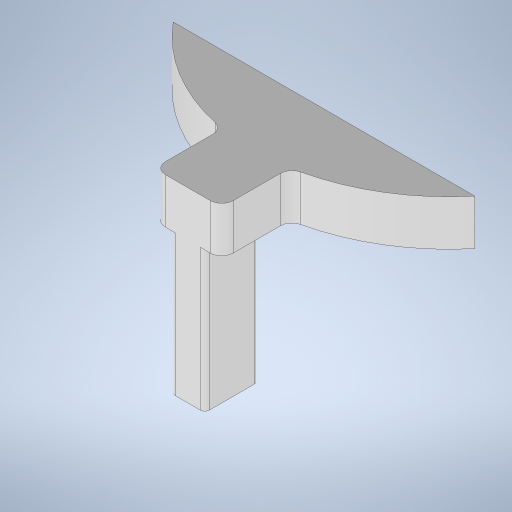
# Autodesk Inventor part: zigu1
Saved by Autodesk Inventor 2024.3 (Build 283343010, 343A)
## iProperties
Created: 2025-10-17
Part Number: zigu1
Material: 一般
Document SubType Name: Modeling
Designer: tanoue_kota
Density: 1 g/cm^3
Appearance: 既定
Author: tanoue_kota
Autodesk Inventor part; units mm, degrees
ref_plane "YZ Plane" through (0, 0, 0) normal (1, 0, 0) x (0, 1, 0)
ref_plane "XZ Plane" through (0, 0, 0) normal (0, 1, 0) x (-1, 0, 0)
ref_plane "XY Plane" through (0, 0, 0) normal (0, 0, 1) x (1, 0, 0)
sketch "スケッチ1" plane through (0, 0, 0) normal (0, 1, 0) x (-1, 0, 0)
  circle A0 centre (0, 0) radius 86.2565
  line L0 (0, 0) -> (86.2565, 0)
  line L1 (66.4468, 55) -> (-66.4468, 55)
  line L2 (0, 55) -> (14.9, 55)
  line L3 (14.9, 55) -> (14.9, 115)
  line L4 (14.9, 115) -> (0, 115)
  line L5 (0, 115) -> (0, 55)
  line L6 (-14.9, 55) -> (-14.9, 115)
  line L7 (-14.9, 115) -> (0, 115)
  point P0 (14.9, 84.9598)
  point P1 (-14.9, 84.9598)
  dimension "d0" = 172.513
  dimension "d1" = 55
  dimension "d2" = 14.9
  dimension "d3" = 60
  constraints: 16 end point, 3 parallel, 3 point on circle, 2 horizontal, 2 symmetric about line, 1 centre point, 1 coincident, 1 midpoint, 1 perpendicular
  measures "d0" diameter of A0
  measures "d1" distance between parallel lines of L0 L1
  measures "d2" distance between parallel lines of L5 L3
  measures "d3" distance between parallel lines of L1 L4
extrude "押し出し1" add sketch "スケッチ1" along normal blind 20 contours L1 L3 A0 | A0 L6 L1 | L3 L1 L5 A0 | A0 L5 L4 L3 | L6 L7 L5 A0 | A0 L5 L1 L6
sketch "スケッチ2" plane through (0, 0, 0) normal (0, -1, 0) x (1, 0, 0)
  arc A0 (66.4468, 55) -> (14.9, 84.9598) centre (0, 0) ccw projected
  circle A1 centre (0, 0) radius 86.2565
  line L0 (-14.9, 115) -> (14.9, 115) projected
  line L1 (0, 115) -> (7.475, 115)
  line L2 (7.475, 115) -> (7.475, 91.2565)
  line L3 (7.475, 91.2565) -> (0, 91.2565)
  line L4 (0, 91.2565) -> (0, 115)
  line L5 (-7.475, 115) -> (-7.475, 91.2565)
  line L6 (-7.475, 91.2565) -> (0, 91.2565)
  line L7 (14.9, 115) -> (-14.9, 115)
  dimension "d6" = 5
  dimension "d7" = 7.475
  constraints: 14 end point, 4 symmetric about line, 2 parallel, 1 coincident, 1 horizontal, 1 midpoint, 1 perpendicular, 3 other
  measures "d7" distance of L2.end L3.end
extrude "押し出し2" add sketch "スケッチ2" along normal blind 62.1 contours L0 L4 L6 L5 | L0 L2 L3 L4
fillet "フィレット1" radius 5 4 edges at (-14.9, 10, 84.9598) (14.9, 10, 84.9598) (-14.9, 10, 115) (14.9, 10, 115)
fillet "フィレット2" radius 2 4 edges at (-7.475, -31.05, 91.2565) (7.475, -31.05, 91.2565) (-7.475, -31.05, 115) (7.475, -31.05, 115)
